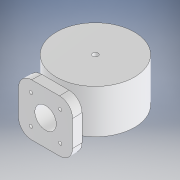
# Autodesk Inventor part: AA035
Saved by Autodesk Inventor 2017 SP1 (Build 210196100, 196)
## iProperties
Created: 2017-10-23
Part Number: AA035
Material: ABS Plastic
Document SubType Name: Modeling
Designer: Zach
Categories: <?xml version="1.0" encoding="UTF-16"?> <MemberInstance><Categories><FamilyTemplate><FamilyTemplateParameter ValueType="xs:double" Id="1" ObjectReferenceKey="da_z" ObjectType="kUserParameterObject"/><FamilyTemplateParameter ValueType="xs:double" Id="2" ObjectReferenceKey="da_b" ObjectType="kUserParameterObject"/><FamilyTemplateParameter ValueType="xs:double" Id="3" ObjectReferenceKey="da_beta" ObjectType="kUserParameterObject"/><FamilyTemplateParameter ValueType="xs:double" Id="4" ObjectReferenceKey="da_da" ObjectType="kUserParameterObject"/><FamilyTemplateParameter ValueType="xs:double" Id="5" ObjectReferenceKey="da_aw" ObjectType="kUserParameterObject"/><FamilyTemplateParameter ValueType="xs:string" Id="6" ObjectReferenceKey="EAIAABAAAACIAQAAAAAAAIAAAAAAAAAA" ObjectType="83910656" SubObjectId="SurfaceGeometry"/></FamilyTemplate><ParamToTemplateMap><ParamToTemplate CategoryParameter="//CategoryParameter[@InternalName='046C89C9-8512-4d59-83FE-43B91F4F132A']" TemplateParameter="1"/><ParamToTemplate CategoryParameter="//CategoryParameter[@InternalName='2552DF32-E462-4b46-AEBF-C6C7768E72AC']" TemplateParameter="2"/><ParamToTemplate CategoryParameter="//CategoryParameter[@InternalName='C9EE641D-15FC-4fae-A226-E94C4372FDD7']" TemplateParameter="3"/><ParamToTemplate><ParamToTemplate CategoryParameter="//CategoryParameter[@InternalName='00B6519A-459B-49c7-AD84-2E56D39A5744']" ConstantValue="0.341447"/></ParamToTemplate><ParamToTemplate><ParamToTemplate CategoryParameter="//CategoryParameter[@InternalName='04B31F0E-C7A6-4894-AA32-9629BEFACF47']" ConstantValue="1.000000"/></ParamToTemplate><ParamToTemplate><ParamToTemplate CategoryParameter="//CategoryParameter[@InternalName='43CBEC2E-7847-49e7-A936-2F7889FCB2D9']" ConstantValue="0.250000"/></ParamToTemplate><ParamToTemplate><ParamToTemplate CategoryParameter="//CategoryParameter[@InternalName='B1EFC894-105D-4ebd-86BF-FA20ED196853']" ConstantValue="0.350000"/></ParamToTemplate><ParamToTemplate><ParamToTemplate CategoryParameter="//CategoryParameter[@InternalName='51175063-3D10-4879-93E8-6246FE8B403D']" ConstantValue="2060000000.000000"/></ParamToTemplate><ParamToTemplate><ParamToTemplate CategoryParameter="//CategoryParameter[@InternalName='A3A52E27-4454-46a9-B0BD-C932399B70AF']" ConstantValue="0.300000"/></ParamToTemplate><ParamToTemplate><ParamToTemplate CategoryParameter="//CategoryParameter[@InternalName='91B76062-C214-41d9-B1B9-14D2AB99603D']" ConstantValue="0.200000"/></ParamToTemplate><ParamToTemplate><ParamToTemplate CategoryParameter="//CategoryParameter[@InternalName='374E806E-8B8A-4dda-A9AA-1039D6500AD2']" ConstantValue="5.000000"/></ParamToTemplate><ParamToTemplate><ParamToTemplate CategoryParameter="//CategoryParameter[@InternalName='2D373A89-B862-43d6-8D0B-0CBF12AB9F6C']" ConstantValue="0.392699"/></ParamToTemplate><ParamToTemplate CategoryParameter="//CategoryParameter[@InternalName='37777632-D6A2-4fac-9D53-DB8ACD95C989']" TemplateParameter="4"/><ParamToTemplate CategoryParameter="//CategoryParameter[@InternalName='FD1017F1-B727-4f7e-9707-0F86F1FF9423']" TemplateParameter="5"/><ParamToTemplate><ParamToTemplate CategoryParameter="//CategoryParameter[@InternalName='9E1B4470-B2D3-4ff1-B813-535BB4CDF51A']" ConstantValue="3520000.000000"/></ParamToTemplate><ParamToTemplate><ParamToTemplate CategoryParameter="//CategoryParameter[@InternalName='F8452263-BFF6-458c-9FB1-07C4B99E95CD']" ConstantValue="11400000.000000"/></ParamToTemplate><ParamToTemplate><ParamToTemplate CategoryParameter="//CategoryParameter[@InternalName='3E3BB259-FD49-497f-8171-6EBC954A3479']" ConstantValue="2.000000"/></ParamToTemplate><ParamToTemplate CategoryParameter="//CategoryParameter[@InternalName='27C3BAF2-7550-4e4b-AE2C-0DB134B7D9B7']" TemplateParameter="6"/></ParamToTemplateMap><Category DisplayName="Gear" InternalName="DC85795E-93AB-48d5-8EEE-5A27447B64BD" Mnemonic="Gear"><CategoryParameter DisplayName="z" InternalName="046C89C9-8512-4d59-83FE-43B91F4F132A" Mnemonic="z"/><CategoryParameter DisplayName="b" InternalName="2552DF32-E462-4b46-AEBF-C6C7768E72AC" Mnemonic="b"/><CategoryParameter DisplayName="||b|" InternalName="C9EE641D-15FC-4fae-A226-E94C4372FDD7" Mnemonic="beta"/><CategoryParameter DisplayName="x" InternalName="00B6519A-459B-49c7-AD84-2E56D39A5744" Mnemonic="x"/><CategoryParameter DisplayName="a*" InternalName="04B31F0E-C7A6-4894-AA32-9629BEFACF47" Mnemonic="a"/><CategoryParameter DisplayName="c*" InternalName="43CBEC2E-7847-49e7-A936-2F7889FCB2D9" Mnemonic="c"/><CategoryParameter DisplayName="r|.f|*" InternalName="B1EFC894-105D-4ebd-86BF-FA20ED196853" Mnemonic="rf"/><CategoryParameter DisplayName="E" InternalName="51175063-3D10-4879-93E8-6246FE8B403D" Mnemonic="E"/><CategoryParameter DisplayName="||m|" InternalName="A3A52E27-4454-46a9-B0BD-C932399B70AF" Mnemonic="mi"/><Category DisplayName="SpurGear" InternalName="26C5A22E-A91E-4dfd-A3B3-23CCAFAE1764" Mnemonic="SpurGear"><CategoryParameter DisplayName="m" InternalName="91B76062-C214-41d9-B1B9-14D2AB99603D" Mnemonic="m"/><CategoryParameter DisplayName="P" InternalName="374E806E-8B8A-4dda-A9AA-1039D6500AD2" Mnemonic="PP"/><CategoryParameter DisplayName="||a|" InternalName="2D373A89-B862-43d6-8D0B-0CBF12AB9F6C" Mnemonic="alpha"/><CategoryParameter DisplayName="d|.a|" InternalName="37777632-D6A2-4fac-9D53-DB8ACD95C989" Mnemonic="da"/><CategoryParameter DisplayName="a|.w|" InternalName="FD1017F1-B727-4f7e-9707-0F86F1FF9423" Mnemonic="aw"/><CategoryParameter DisplayName="||s||.Flim|" InternalName="9E1B4470-B2D3-4ff1-B813-535BB4CDF51A" Mnemonic="sFlim"/><CategoryParameter DisplayName="||s||.Hlim|" InternalName="F8452263-BFF6-458c-9FB1-07C4B99E95CD" Mnemonic="sHlim"/><CategoryParameter DisplayName="type" InternalName="3E3BB259-FD49-497f-8171-6EBC954A3479" Mnemonic="type"/><CategoryParameter DisplayName="PitchDiameter" InternalName="27C3BAF2-7550-4e4b-AE2C-0DB134B7D9B7" Mnemonic="IDS_PITCHDIAM"/></Category></Category></Categories></MemberInstance>
Density: 1.06 g/cm^3
Appearance: CR White
CustomPartVersion: 1
Author: Zach
Autodesk Inventor part; units mm, degrees
ref_plane "YZ Plane" through (0, 0, 0) normal (1, 0, 0) x (0, 1, 0)
ref_plane "XZ Plane" through (0, 0, 0) normal (0, 1, 0) x (-1, 0, 0)
ref_plane "XY Plane" through (0, 0, 0) normal (0, 0, 1) x (1, 0, 0)
sketch "Sketch1" plane through (0, 0, 0) normal (0, 0, 1) x (1, 0, 0)
  circle A0 centre (0, 0) radius 60.406
  dimension "d0" = 120.812
  constraints: 1 centre point
  measures "d0" diameter of A0
extrude "Extrusion1" add sketch "Sketch1" along normal blind 12.5
ref_plane "Work Plane2" through (0, 0, 6.25) normal (0, 0, 1) x (1, 0, 0)
sketch "Sketch2" plane through (0, 0, 0) normal (0, 0, -1) x (-1, 0, 0)
  circle A0 centre (0, 0) radius 60.406 projected
  circle A1 centre (0, 0) radius 58.2143
  dimension "d3" = 116.4286
  constraints: 1 centre point, 1 coincident
  measures "d3" diameter of A1
surface extrude "Pitch Diameter" sketch "Sketch2" against normal through all shown no curves A1
ref_plane "Work Plane8" through (0, 0, 0) normal (0.9980267, 0.0627905, 0) x (0, 0, 1)
ref_plane "Work Plane9" through (0, 0, 0) normal (1, 0, 0) x (0, 1, 0)
spur gear teeth "Spur Gear" teeth 50 pitch diameter 115.4701 tip diameter 120.812 root diameter 111.8358 face width 12.5 helix angle 30 hand right start plane through (0, 0, 0) normal (0, 0, -1) x (-1, 0, 0)
mirror "Mirror1" about plane through (0, 0, 12.5) normal (0, 0, 1)
sketch "Sketch3" plane through (0, 0, 25) normal (0, 0, 1) x (0.9685832, 0.2486899, 0)
  circle A0 centre (0, 0) radius 60
  dimension "d49" = 120
  constraints: 1 centre point, 1 coincident
  measures "d49" diameter of A0
extrude "Extrusion2" add sketch "Sketch3" along normal blind 67
sketch "Sketch4" plane through (0, 0, 92) normal (0, 0, 1) x (1, 0, 0)
  circle A0 centre (0, 0) radius 4.25
  dimension "d52" = 8.5
  constraints: 1 centre point, 1 coincident
  measures "d52" diameter of A0
extrude "Extrusion3" cut sketch "Sketch4" against normal through all
ref_plane "Work Plane11" through (0, 0, 46) normal (0, 0, 1) x (1, 0, 0)
sketch "Sketch6" plane through (0, 0, 46) normal (0, 0, 1) x (1, 0, 0)
  line L0 (-25, -54.5436) -> (25, -54.5436)
  line L1 (25, -54.5436) -> (25, -61.5436)
  line L2 (25, -61.5436) -> (-25, -61.5436)
  line L3 (-25, -61.5436) -> (-25, -54.5436)
  circle A0 centre (0, 0) radius 4.25 construction
  circle A1 centre (0, 0) radius 60 construction
  dimension "d63" = 50
  dimension "d64" = 7
  constraints: 8 end point, 2 parallel, 2 point on circle, 1 horizontal, 1 perpendicular
  measures "d63" distance of L1.end L2.end
  measures "d64" distance of L0.end L1.end
extrude "Extrusion5" add sketch "Sketch6" along normal mid plane 42
sketch "Sketch7" plane through (0, 0, 46) normal (0, 0, 1) x (1, 0, 0)
  line L0 (-41, -61.5436) -> (41, -61.5436)
  line L1 (41.5215, -76.5436) -> (-41.5215, -76.5436)
  line L2 (25, -61.5436) -> (-25, -61.5436) projected
  line L3 (-41.5215, -76.5436) -> (-41, -61.5436)
  line L4 (41.5215, -76.5436) -> (41, -61.5436)
  point P0 (0, 0)
  point P1 (0, -61.5436)
  point P2 (0, -76.5436)
  dimension "d67" = 83.043
  dimension "d99" = 82
  dimension "d100" = 15
  constraints: 8 end point, 3 midpoint, 1 horizontal, 1 parallel, 1 vertical alignment
  measures "d67" distance of L1.start L1.end
  measures "d99" distance of L0.start L0.end
  measures "d100" distance between parallel lines of L0 L1
extrude "Extrusion6" add sketch "Sketch7" along normal mid plane 80
sketch "Sketch8" plane through (-41.5215, -76.5436, 86) normal (0, -1, 0) x (1, 0, 0)
  line L0 (64.0215, -62.5) -> (19.0215, -62.5) construction
  line L1 (19.0215, -62.5) -> (19.0215, -17.5) construction
  line L2 (19.0215, -17.5) -> (64.0215, -17.5) construction
  line L3 (64.0215, -17.5) -> (64.0215, -62.5) construction
  circle A0 centre (64.0215, -62.5) radius 2.5
  circle A1 centre (64.0215, -17.5) radius 2.5
  circle A2 centre (19.0215, -62.5) radius 2.5
  circle A3 centre (19.0215, -17.5) radius 2.5
  line L4 (0, 0) -> (83.043, 0) projected
  line L5 (83.043, 0) -> (83.043, -80) projected
  point P0 (23.25, -86)
  point P1 (41.5215, -17.5)
  point P2 (41.5215, 0)
  point P3 (64.0215, -40)
  point P4 (83.043, -40)
  dimension "d75" = 45
  dimension "d78" = 5
  dimension "d79" = 5
  dimension "d101" = 45
  dimension "d102" = 5
  dimension "d103" = 5
  constraints: 8 end point, 4 centre point, 4 coincident, 4 midpoint, 2 parallel, 1 horizontal, 1 horizontal alignment, 1 perpendicular, 1 vertical alignment
  measures "d75" distance of L0.end L1.end
  measures "d78" diameter of A2
  measures "d79" diameter of A3
  measures "d101" distance of L1.end L2.end
  measures "d102" diameter of A1
  measures "d103" diameter of A0
extrude "Extrusion7" cut sketch "Sketch8" against normal blind 25
sketch "Sketch9" plane through (-41.5215, -76.5436, 86) normal (0, -1, 0) x (1, 0, 0)
  circle A0 centre (41.5215, -40) radius 16.5
  circle A1 centre (19.0215, -62.5) radius 2.5 construction
  circle A2 centre (64.0215, -62.5) radius 2.5 construction
  circle A3 centre (64.0215, -17.5) radius 2.5 construction
  circle A4 centre (19.0215, -17.5) radius 2.5 construction
  line L0 (83.043, 0) -> (83.043, -80) construction
  line L1 (0, 0) -> (83.043, 0) construction
  line L2 (0, 0) -> (0, -80) construction
  line L3 (83.043, -80) -> (0, -80) construction
  point P0 (23.25, -86)
  point P1 (0, -40)
  point P2 (41.5215, 0)
  dimension "d82" = 33
  constraints: 2 midpoint, 1 centre point, 1 horizontal alignment, 1 vertical alignment
  measures "d82" diameter of A0
extrude "Extrusion8" cut sketch "Sketch9" against normal blind 45
sketch "Sketch14" plane through (0, 0, 46) normal (0, 0, 1) x (1, 0, 0)
  line L0 (16.5, -76.5436) -> (16.5, -31.5436) projected
  line L1 (16.5, -31.5436) -> (-16.5, -31.5436)
  line L2 (-16.5, -31.5436) -> (-16.5, -16.5436)
  line L3 (-16.5, -16.5436) -> (16.5, -16.5436)
  line L4 (16.5, -16.5436) -> (16.5, -31.5436)
  point P0 (0, 0)
  dimension "d91" = 33
  dimension "d92" = 15
  constraints: 8 end point, 2 parallel, 1 horizontal, 1 perpendicular
  measures "d91" distance of L2.end L3.end
  measures "d92" distance of L1.end L2.end
extrude "Extrusion10" cut sketch "Sketch14" along normal mid plane 33
sketch "Sketch15" plane through (16.5, -31.5436, 29.5) normal (-1, 0, 0) x (0, 0, 1)
  line L0 (33, 15) -> (0, 15) projected
  line L1 (0, 15) -> (0, 0) projected
  line L2 (0, 0) -> (16.5, 0) projected
  line L3 (16.5, 0) -> (33, 0) projected
  line L4 (33, 0) -> (33, 15) projected
  line L5 (21.5, 12.5) -> (11.5, 12.5)
  line L6 (11.5, 12.5) -> (11.5, 2.5)
  line L7 (11.5, 2.5) -> (21.5, 2.5)
  line L8 (21.5, 2.5) -> (21.5, 12.5)
  point P0 (-29.5, 31.5436)
  point P1 (16.5, 2.5)
  point P2 (21.5, 7.5)
  point P3 (33, 7.5)
  dimension "d95" = 10
  dimension "d96" = 10
  constraints: 8 end point, 3 midpoint, 2 parallel, 1 horizontal, 1 horizontal alignment, 1 perpendicular, 1 vertical alignment
  measures "d95" distance of L7.end L6.end
  measures "d96" distance of L6.end L5.end
extrude "Extrusion11" cut sketch "Sketch15" along normal through all contours L8 L7 L6 L5
fillet "Fillet4" radius 20 4 edges at (41.2608, -69.0436, 86) (41.2608, -69.0436, 6) (-41.2608, -69.0436, 86) (-41.2608, -69.0436, 6)
sketch "Sketch16" plane through (0, 0, 25) normal (0, 0, -1) x (-0.9685832, -0.2486899, 0)
  circle A0 centre (0, 0) radius 60 projected
  circle A1 centre (0, 0) radius 63
  dimension "d107" = 3
  constraints: 1 centre point
  measures "d107" radial gap between concentric circles of A0 A1
extrude "Extrusion12" cut sketch "Sketch16" along normal through all contours A0 | A1
sketch "Sketch17" plane through (0, 0, 25) normal (0, 0, -1) x (-0.9685832, -0.2486899, 0)
  circle A0 centre (33.9004, 8.7041) radius 2.5
  circle A1 centre (9.4122, 33.7107) radius 2.5
  circle A2 centre (-24.4882, 25.0065) radius 2.5
  circle A3 centre (-33.9004, -8.7041) radius 2.5
  circle A4 centre (-9.4122, -33.7107) radius 2.5
  circle A5 centre (24.4882, -25.0065) radius 2.5
  line L0 (33.9004, 8.7041) -> (-33.9004, -8.7041) construction
  line L1 (-1.7981, -79.488) -> (39.8693, -68.7896) projected
  point P0 (0, 0)
  dimension "d108" = 5
  dimension "d109" = 35
  dimension "d112" = 360
  constraints: 6 centre point, 2 end point, 1 parallel, 13 other
  measures "d108" diameter of A0
  measures "d109" distance of point (0, 0) L0.start
extrude "Extrusion13" cut sketch "Sketch17" against normal blind 25
equation "\"d0\" = da_da"
equation "\"d1\" = da_b"
equation "\"d3\" = da_dw"
equation "\"d16\" = da_aw"
equation "\"d43\" = da_aw"
equation "\"d46\" = da_aw"
equation "\"da_da\" = 120.811978"
equation "\"da_b\" = 12.5"
equation "\"da_dw\" = 116.428571"
equation "\"da_aw\" = 81.5"
body "Solid1"
body "Srf1"
